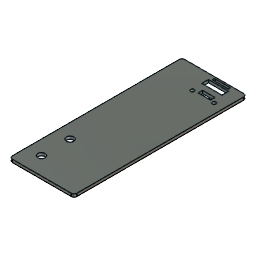
z_stop (Autodesk Fusion 360 design; units mm, degrees)
Autodesk Fusion 360 part; units mm, degrees
sketch "Esboço1" plane through (0, 0, 0) normal (0, 0, 1) x (1, 0, 0)
  line L0 (-20.5, 60) -> (20.5, 60)
  line L1 (22.5, 58) -> (22.5, -58)
  line L2 (20.5, -60) -> (-20.5, -60)
  line L3 (-22.5, -58) -> (-22.5, 58)
  line L4 (-22.5, 60) -> (22.5, -60) construction
  line L5 (22.5, 60) -> (-22.5, -60) construction
  arc A0 (20.5, -60) -> (22.5, -58) centre (20.5, -58) ccw
  arc A1 (22.5, 58) -> (20.5, 60) centre (20.5, 58) ccw
  arc A2 (-20.5, 60) -> (-22.5, 58) centre (-20.5, 58) ccw
  arc A3 (-22.5, -58) -> (-20.5, -60) centre (-20.5, -58) ccw
  dimension "d1" = 45
  dimension "d2" = 120
  dimension "d27" = 2
  constraint horizontal L0
  constraint perpendicular L0 L1
  constraint parallel L0 L2
  constraint parallel L1 L3
  constraint coincident L4 origin
  constraint coincident L5 origin
  constraint coincident L4.end L2
  constraint coincident L4.end L1
  constraint tangent L2 A0
  constraint tangent L1 A0
  constraint coincident L5.start L0
  constraint coincident L5.start L1
  constraint tangent L0 A1
  constraint tangent L1 A1
  constraint equal A0 A1
  constraint coincident L4.start L3
  constraint coincident L4.start L0
  constraint tangent L3 A2
  constraint tangent L0 A2
  constraint equal A0 A2
  constraint coincident L5.end L2
  constraint coincident L5.end L3
  constraint tangent L2 A3
  constraint tangent L3 A3
  constraint equal A0 A3
  measures "d1" distance of L4.end L5.end
  measures "d2" distance of L5.start L4.end
  measures "d27" radius of A0
extrude "Extrusão1" add sketch "Esboço1" along normal blind 2
sketch "Esboço2" plane through (0, 0, 2) normal (0, 0, 1) x (-1, 0, 0)
  line L0 (20.5, 60) -> (-20.5, 60)
  line L1 (-22.5, 58) -> (-22.5, -58)
  line L2 (-20.5, -60) -> (20.5, -60)
  line L3 (22.5, -58) -> (22.5, 58)
  circle A0 centre (12.45, 27.78) radius 2.55
  circle A1 centre (12.45, 47.65) radius 2.55
  line L4 (0.19, -51.5) -> (-13.81, -51.5)
  line L5 (-13.81, -51.5) -> (-13.81, -56.1)
  line L6 (-13.81, -56.1) -> (0.19, -56.1)
  line L7 (0.19, -56.1) -> (0.19, -51.5)
  line L8 (0.19, -51.5) -> (-13.81, -56.1) construction
  line L9 (-13.81, -51.5) -> (0.19, -56.1) construction
  line L10 (-4.26, -44.55) -> (-12.86, -44.55)
  line L11 (-12.86, -44.55) -> (-12.86, -47.55)
  line L12 (-12.86, -47.55) -> (-4.26, -47.55)
  line L13 (-4.26, -47.55) -> (-4.26, -44.55)
  line L14 (-4.26, -44.55) -> (-12.86, -47.55) construction
  line L15 (-12.86, -44.55) -> (-4.26, -47.55) construction
  circle A2 centre (-0.76, -43.98) radius 1.25
  circle A3 centre (-15.86, -43.98) radius 1.25
  arc A4 (20.5, -60) -> (22.5, -58) centre (20.5, -58) ccw
  arc A5 (22.5, 58) -> (20.5, 60) centre (20.5, 58) ccw
  arc A6 (-20.5, 60) -> (-22.5, 58) centre (-20.5, 58) ccw
  arc A7 (-22.5, -58) -> (-20.5, -60) centre (-20.5, -58) ccw
  line L16 (-1.81, -57.3) -> (-11.81, -57.3)
  arc A8 (-11.81, -57.3) -> (-11.81, -58.8) centre (-11.81, -58.05) ccw
  line L17 (-11.81, -58.8) -> (-1.81, -58.8)
  arc A9 (-1.81, -58.8) -> (-1.81, -57.3) centre (-1.81, -58.05) ccw
  line L18 (-1.81, -58.05) -> (-11.81, -58.05) construction
  point P0 (-6.81, -53.8)
  point P1 (-8.56, -46.05)
  dimension "d5" = 5.1
  dimension "d6" = 5.1
  dimension "d7" = 19.87
  dimension "d8" = 10.05
  dimension "d9" = 10.05
  dimension "d11" = 14
  dimension "d12" = 4.6
  dimension "d13" = 8.6
  dimension "d14" = 3
  dimension "d15" = 9.64
  dimension "d16" = 8.69
  dimension "d17" = 3.95
  dimension "d18" = 3.9
  dimension "d19" = 2.5
  dimension "d20" = 2.5
  dimension "d21" = 15.1
  dimension "d22" = 6.64
  dimension "d23" = 16.02
  dimension "d24" = 16.02
  dimension "d29" = 12.35
  dimension "d30" = 1.5
  dimension "d31" = 10
  constraint horizontal L4
  constraint perpendicular L4 L5
  constraint parallel L4 L6
  constraint parallel L5 L7
  constraint coincident L8 P0
  constraint coincident L9 P0
  constraint horizontal L10
  constraint perpendicular L10 L11
  constraint parallel L10 L12
  constraint parallel L11 L13
  constraint coincident L14 P1
  constraint coincident L15 P1
  constraint tangent L16 A8
  constraint tangent A8 L17
  constraint parallel L16 L17
  constraint tangent L17 A9
  constraint tangent L16 A9
  measures "d5" diameter of A0
  measures "d6" diameter of A1
  measures "d7" vertical distance of A0.centre A1.centre
  measures "d8" distance of L3 A1.centre
  measures "d9" distance of L3 A0.centre
  measures "d11" distance of L5.end L6.end
  measures "d12" distance of L4.end L5.end
  measures "d13" distance of L11.end L12.end
  measures "d14" distance of L10.end L11.end
  measures "d15" distance of L1 L11
  measures "d16" distance of L1 L5
  measures "d17" distance of L4 L12
  measures "d18" distance of L2 L6
  measures "d19" diameter of A2
  measures "d20" diameter of A3
  measures "d21" distance of A2.centre A3.centre
  measures "d22" distance of L1 A3.centre
  measures "d23" distance of L2 A3.centre
  measures "d24" distance of L2 A2.centre
  measures "d29" distance of L0 A1.centre
  measures "d30" diameter of A8
  measures "d31" distance of A9.centre A8.centre
extrude "Extrusão2" cut sketch "Esboço2" against normal blind 15 contours A0 | A1 | L4 L5 L6 L7 | L10 L11 L12 L13 | A2 | A3 | L16 A8 L17 A9
sketch "Esboço4" plane through (0, 0, 2) normal (0, 0, 1) x (-1, 0, 0)
  circle A0 centre (12.45, 27.78) radius 2.55
  circle A1 centre (-15.86, -43.98) radius 1.25
  circle A2 centre (-0.76, -43.98) radius 1.25
  circle A3 centre (12.45, 47.65) radius 2.55
  line L0 (-12.86, -44.55) -> (-4.26, -44.55)
  line L1 (-4.26, -44.55) -> (-4.26, -47.55)
  line L2 (-4.26, -47.55) -> (-12.86, -47.55)
  line L3 (-12.86, -47.55) -> (-12.86, -44.55)
  line L4 (-13.81, -51.5) -> (0.19, -51.5)
  line L5 (0.19, -51.5) -> (0.19, -56.1)
  line L6 (0.19, -56.1) -> (-13.81, -56.1)
  line L7 (-13.81, -56.1) -> (-13.81, -51.5)
  line L8 (-11.81, -57.3) -> (-1.81, -57.3)
  arc A4 (-1.81, -58.8) -> (-1.81, -57.3) centre (-1.81, -58.05) ccw
  line L9 (-1.81, -58.8) -> (-11.81, -58.8)
  arc A5 (-11.81, -57.3) -> (-11.81, -58.8) centre (-11.81, -58.05) ccw
  arc A6 (20.5, -60) -> (22.5, -58) centre (20.5, -58) ccw
  line L10 (22.5, -58) -> (22.5, 58)
  arc A7 (22.5, 58) -> (20.5, 60) centre (20.5, 58) ccw
  line L11 (20.5, 60) -> (-20.5, 60)
  arc A8 (-20.5, 60) -> (-22.5, 58) centre (-20.5, 58) ccw
  line L12 (-22.5, 58) -> (-22.5, -58)
  arc A9 (-22.5, -58) -> (-20.5, -60) centre (-20.5, -58) ccw
  line L13 (-20.5, -60) -> (20.5, -60)
equation "d15 = 5.25 mm + 4.39 mm"
equation "d16 = 4.3 mm + 4.39 mm"
equation "d22 = 2.25 mm + 4.39 mm"
